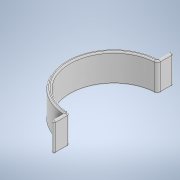
# Autodesk Inventor part: handle
Saved by Autodesk Inventor 2020 (Build 240168000, 168)
## iProperties
Created: 2020-06-27
Part Number: handle
Material: Generic
Document SubType Name: Modeling
Designer: maple
Density: 1 g/cm^3
Appearance: Default
Author: maple
Autodesk Inventor part; units mm, degrees
ref_plane "YZ Plane" through (0, 0, 0) normal (1, 0, 0) x (0, 1, 0)
ref_plane "XZ Plane" through (0, 0, 0) normal (0, 1, 0) x (-1, 0, 0)
ref_plane "XY Plane" through (0, 0, 0) normal (0, 0, 1) x (1, 0, 0)
sketch "Sketch1" plane through (0, 0, 0) normal (0, 1, 0) x (-1, 0, 0)
  line L0 (0, 0) -> (0, -100)
  line L1 (0, -50) -> (50, -50)
  circle A0 centre (0, -50) radius 50
  line L2 (50, -50) -> (46, -50)
  line L3 (0, 0) -> (0, 13)
  line L4 (0, -100) -> (0, -113)
  circle A1 centre (0, -50) radius 46
  line L5 (0, 13) -> (3, 13)
  line L6 (3, 13) -> (3, -0.99065)
  line L7 (3, -0.99065) -> (0, -0.99065)
  line L8 (0, -0.99065) -> (0, 13)
  line L9 (0, -113) -> (3, -113)
  line L10 (3, -113) -> (3, -98.99687)
  line L11 (3, -98.99687) -> (0, -98.99687)
  line L12 (0, -98.99687) -> (0, -113)
  point P0 (0, -4)
  point P1 (0, -96)
  point P2 (3, -99.909919)
  point P3 (3, -0.090081)
  dimension "d0" = 100
  dimension "d1" = 50
  dimension "d2" = 4
  dimension "d3" = 13
  dimension "d4" = 13
  dimension "d5" = 3
  dimension "d6" = 3
  constraints: 26 end point, 4 parallel, 3 horizontal, 3 vertical, 2 coincident, 2 perpendicular, 1 midpoint, 1 point on line, 6 other
  measures "d0" distance of L0.start L0.end
  measures "d1" distance of L1.start L1.end
  measures "d2" distance of L1.end L2.end
  measures "d3" distance of L0.start L3.end
  measures "d4" distance of L0.end L4.end
  measures "d5" distance of L6.end L7.end
  measures "d6" distance of L11.end L10.end
sketch "Sketch1 outline for Extrusion1" plane through (0, 0, 0) normal (0, 1, 0) x (-1, 0, 0)
  line L0 (3, 13) -> (0, 13)
  line L1 (3, -0.090081) -> (3, 13)
  arc A0 (3, -99.909919) -> (3, -0.090081) centre (0, -50) ccw
  line L2 (3, -113) -> (3, -99.909919)
  line L3 (0, -113) -> (3, -113)
  line L4 (0, -100) -> (0, -113)
  line L5 (0, -96) -> (0, -100)
  arc A1 (0, -4) -> (0, -96) centre (0, -50) cw
  line L6 (0, 0) -> (0, -4)
  line L7 (0, 13) -> (0, 0)
extrude "Extrusion1" add sketch "Sketch1 outline for Extrusion1" along normal blind 30
fillet "Fillet1" radius 3.175 2 edges at (0, 15, -96) (0, 15, -4)
fillet "Fillet2" radius 1.5 4 edges at (-3, 15, 13) (0, 15, 13) (-3, 15, -113) (0, 15, -113)
fillet "Fillet3" radius 1.5 20 edges at (-0.8586, 30, -96.901) (-0.8586, 30, -3.099) (0, 30, -99.5362) (0, 30, -0.4638) (-2.5607, 30, -112.5607) (-3, 30, -105.705) (-2.5607, 30, 12.5607) (-3, 30, 5.705) (-46, 30, -50) (-50, 30, -50) (-0.8586, 0, -96.901) (-0.8586, 0, -3.099) (0, 0, -99.5362) (0, 0, -0.4638) (-2.5607, 0, -112.5607) (-3, 0, -105.705) (-2.5607, 0, 12.5607) (-3, 0, 5.705) (-46, 0, -50) (-50, 0, -50)
body "Solid1"
